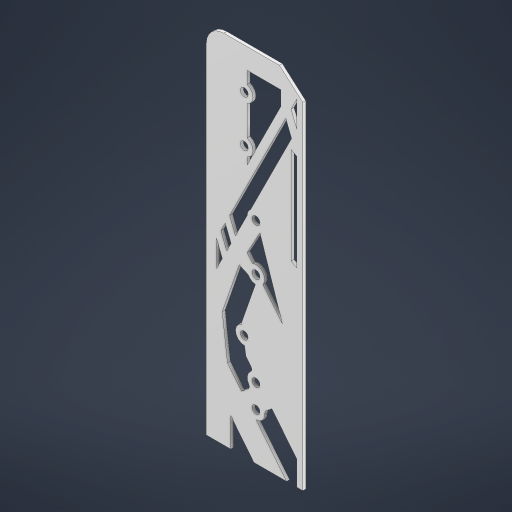
# Autodesk Inventor part: sideplate
Saved by Autodesk Inventor 2024 (Build 280153000, 153)
## iProperties
Created: 2023-11-07
Part Number: sideplate
Material: Acetal Resin, White
Document SubType Name: Sheet Metal
Designer: avere
Density: 1.425 g/cm^3
Appearance: Smooth - White
Flat Pattern Width: 5.23875 cm
Flat Pattern Length: 19.3675 cm
Flat Pattern Area: 101.461 cm^2
Sheet Metal Rule: Default_mm
Sheet Metal Width: 2.063 in
Sheet Metal Length: 7.625 in
Sheet Metal Area: 15.727 in^2
Author: avere
Autodesk Inventor part; units mm, degrees
ref_plane "YZ Plane" through (0, 0, 0) normal (1, 0, 0) x (0, 1, 0)
ref_plane "XZ Plane" through (0, 0, 0) normal (0, 1, 0) x (-1, 0, 0)
ref_plane "XY Plane" through (0, 0, 0) normal (0, 0, 1) x (1, 0, 0)
sketch "Sketch1" plane through (0, 0, 0) normal (0, 0, 1) x (1, 0, 0)
  circle A0 centre (-1.6749, 21.9538) radius 2.1844
  circle A1 centre (-1.6749, -3.4462) radius 2.1844
  line L0 (23.7251, 85.917) -> (23.7251, -92.3462)
  line L1 (-28.6624, -92.3462) -> (-28.6624, 91.8038)
  line L2 (17.3751, 64.8163) -> (20.5501, 63.2288)
  line L3 (20.5501, 63.2288) -> (20.5501, 10.8413)
  line L4 (20.5501, 10.8413) -> (17.3751, 12.4288)
  line L5 (17.3751, 12.4288) -> (17.3751, 64.8163)
  line L6 (20.5501, 75.9288) -> (17.3751, 83.8663)
  line L7 (20.5501, 90.2163) -> (20.5501, 75.9288)
  line L8 (17.6728, 70.1741) -> (14.4978, 78.1116)
  line L9 (17.3751, 83.8663) -> (20.5501, 90.2163)
  line L10 (-18.3436, 12.4288) -> (-15.1686, 4.4913)
  line L11 (-15.9624, 17.1913) -> (-12.7874, 9.2538)
  line L12 (-15.9624, 17.1913) -> (14.4978, 78.1116)
  line L13 (-23.1061, 2.9038) -> (-19.9311, -5.0337)
  line L14 (-23.1061, 2.9038) -> (-23.1061, -11.3837)
  line L15 (-20.7249, 7.6663) -> (-18.3436, 12.4288)
  line L16 (-15.1686, 4.4913) -> (-17.5499, -0.2712)
  line L17 (-19.9311, -5.0337) -> (-23.1061, -11.3837)
  line L18 (11.8546, 90.2163) -> (11.8546, 82.3502)
  line L19 (11.8546, 90.2163) -> (-6.4374, 90.2163)
  line L20 (11.8546, 82.3502) -> (-6.4374, 45.7663)
  line L21 (0.5095, 17.1913) -> (-6.4374, 4.4913)
  line L22 (12.6126, -19.3212) -> (0.5095, 17.1913)
  line L23 (-10.761, -3.4129) -> (-19.992, -30.0754)
  line L24 (-19.992, -30.0754) -> (-17.153, -52.6587)
  line L25 (-17.153, -52.6587) -> (-9.533, -62.1837)
  line L26 (-9.533, -30.0754) -> (-1.9594, -8.2002)
  line L27 (-5.9563, -5.5321) -> (-10.761, -3.4129)
  line L28 (20.5501, -79.2004) -> (20.5501, -92.3462)
  line L29 (6.9368, -62.1837) -> (4.2652, -64.3209)
  line L30 (-1.5433, -71.7065) -> (14.9685, -92.3462)
  arc A2 (-1.5433, -71.7065) -> (3.0742, -66.8586) centre (-1.6875, -66.9462) ccw
  circle A3 centre (-1.6875, -66.9462) radius 2.1844
  arc A4 (4.2652, -64.3209) -> (3.0742, -66.8586) centre (6.2486, -66.8002) ccw
  line L31 (20.5501, -79.2004) -> (6.9368, -62.1837)
  line L32 (23.7251, -92.3462) -> (20.5501, -92.3462)
  circle A5 centre (-1.6749, -54.2462) radius 2.1844
  arc A6 (-4.5442, -50.4451) -> (-5.5294, -57.0433) centre (-1.6749, -54.2462) ccw
  line L33 (-9.533, -62.1837) -> (-5.8225, -59.2153)
  line L34 (0.5075, -54.1513) -> (0.5095, -54.1497)
  line L35 (0.5095, -54.1497) -> (0.5073, -54.1469)
  line L36 (-4.2611, -48.1864) -> (-7.1105, -44.6247)
  arc A7 (-4.5442, -50.4451) -> (-4.2611, -48.1864) centre (-5.5007, -49.1781) ccw
  arc A8 (-5.8225, -59.2153) -> (-5.5294, -57.0433) centre (-6.8142, -57.9757) ccw
  arc A9 (-4.5324, 25.7638) -> (-6.4374, 21.9538) centre (-1.6749, 21.9538) ccw
  line L37 (17.6728, 70.1741) -> (-4.5324, 25.7638)
  line L38 (-6.4374, 21.9538) -> (-12.7874, 9.2538)
  line L39 (-6.4374, 4.4913) -> (-3.5794, 0.9189)
  line L40 (2.1657, -6.2625) -> (12.6126, -19.3212)
  arc A10 (2.1657, -6.2625) -> (-3.5794, 0.9189) centre (-1.6749, -3.4462) ccw
  arc A11 (-5.9563, -5.5321) -> (-1.9594, -8.2002) centre (-1.6749, -3.4462) ccw
  line L41 (14.9685, -92.3462) -> (44.3118, -92.3462) construction
  line L42 (-2.7748, -92.3462) -> (14.9685, -92.3462)
  line L43 (-28.6624, -92.3462) -> (-23.2121, -92.3462)
  line L44 (-18.5725, -92.3462) -> (-28.6624, -92.3462)
  line L45 (-20.7249, 7.6663) -> (-17.5499, -0.2712)
  line L46 (-28.6624, 98.1538) -> (-28.6624, 101.3288)
  line L47 (-19.1374, 101.3288) -> (11.0251, 101.3288)
  line L48 (23.7251, 90.2163) -> (23.7251, 85.917)
  line L49 (11.0251, 101.3288) -> (23.7251, 90.2163)
  arc A12 (-19.1374, 101.3288) -> (-28.6624, 91.8038) centre (-19.1374, 91.8038) ccw
  arc A13 (-6.4374, 74.6137) -> (-6.4374, 83.5939) centre (-8.0249, 79.1038) ccw
  circle A14 centre (-8.0249, 79.1038) radius 2.1844
  line L50 (-6.4374, 90.2163) -> (-6.4374, 83.5939)
  line L51 (-18.5725, -92.3462) -> (-15.3911, -92.3462)
  line L52 (-15.3911, -92.3462) -> (-15.3911, -76.5759)
  line L53 (-15.3911, -76.5759) -> (-2.7748, -92.3462)
  arc A15 (-6.4374, 49.4405) -> (-6.4374, 58.4207) centre (-8.0249, 53.9306) ccw
  circle A16 centre (-8.0249, 53.9306) radius 2.1844
  line L54 (-6.4374, 74.6137) -> (-6.4374, 58.4207)
  line L55 (-6.4374, 49.4405) -> (-6.4374, 45.7663)
  line L56 (-1.6749, -54.2462) -> (17.3751, -54.2462) construction
  circle A17 centre (-8.0249, -35.1962) radius 2.0955
  arc A18 (-9.4376, -30.6481) -> (-7.8877, -39.9567) centre (-8.0249, -35.1962) ccw
  line L57 (-9.4376, -30.6481) -> (-9.533, -30.0754)
  line L58 (-7.1105, -44.6247) -> (-7.8877, -39.9567)
  point P0 (0, 0)
  point P1 (2.838, -65.4627)
  point P2 (-4.4495, -58.1169)
  point P3 (-3.0588, -49.6892)
  dimension "d0" = 4.3688
  dimension "d1" = 4.3688
  dimension "d3" = 9.525
  dimension "d4" = 4.3688
  dimension "d5" = 3.175
  dimension "d6" = 9.525
  dimension "d7" = 1.5875
  dimension "d8" = 9.525
  dimension "d14" = 3.175
  dimension "d15" = 9.525
  dimension "d18" = 9.525
  dimension "d19" = 4.3688
  dimension "d20" = 3.1814
  dimension "d22" = 9.525
  dimension "d23" = 4.3688
  dimension "d27" = 4.191
  dimension "d28" = 9.525
  constraints: 118 end point, 29 point on circle, 21 perpendicular, 19 centre point, 18 parallel, 8 tangent, 7 coincident, 6 point on line, 6 vertical, 4 horizontal, 2 collinear, 1 equal radius, 3 other
  measures "d0" diameter of A0
  measures "d1" diameter of A1
  measures "d3" diameter of A2
  measures "d4" diameter of A3
  measures "d5" radius of A4
  measures "d6" diameter of A6
  measures "d7" radius of A7
  measures "d8" diameter of A9
  measures "d14" distance of L46.start L46.end
  measures "d15" radius of A12
  measures "d18" diameter of A13
  measures "d19" diameter of A14
  measures "d20" distance of L44.start L51.end
  measures "d22" diameter of A15
  measures "d23" diameter of A16
  measures "d27" diameter of A17
  measures "d28" diameter of A18
extrude "Extrusion1" add sketch "Sketch1" along normal blind 1.5875
equation "\"BendRadius\" = Thickness"
equation "\"BendReliefWidth\" = Thickness"
equation "\"BendReliefDepth\" = 0.5 * Thickness"
equation "\"CornerReliefSize\" = 4 * Thickness"
equation "\"MinimumRemnant\" = 2 * Thickness"
equation "\"TransitionRadius\" = BendRadius"
equation "\"JacobiRadiusSize\" = BendRadius"
equation "\"GapSize\" = Thickness"
equation "\"Thickness\" = 1.5875"
body "Solid1"
